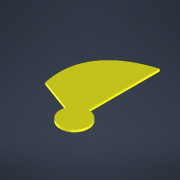
# Autodesk Inventor part: clamshell half
Saved by Autodesk Inventor 2021 (Build 250183000, 183)
## iProperties
Created: 2021-02-13
Part Number: clamshell half
Material: ABS Plastic
Document SubType Name: Modeling
Designer: vikki
Mass: 5.76576 g
Surface Area: 59.2975 cm^2
Volume: 5.43939 cm^3
Density: 1.06 g/cm^3
Appearance: Smooth - Yellow
Author: vikki
Autodesk Inventor part; units mm, degrees
ref_plane "YZ Plane" through (0, 0, 0) normal (1, 0, 0) x (0, 1, 0)
ref_plane "XZ Plane" through (0, 0, 0) normal (0, 1, 0) x (-1, 0, 0)
ref_plane "XY Plane" through (0, 0, 0) normal (0, 0, 1) x (1, 0, 0)
sketch "Sketch1" plane through (0, 0, 0) normal (0, 1, 0) x (-1, 0, 0)
  circle A0 centre (0, 0) radius 12.5
  line L0 (11.7462, -4.2753) -> (40, -14.5588)
  line L1 (0, 0) -> (41.7481, 0) construction
  line L2 (0, 0) -> (11.7462, -4.2753) construction
  line L3 (0, 0) -> (0, -75)
  line L4 (0, -75) -> (27.0598, -66.8927) construction
  line L5 (27.0598, -66.8927) -> (47.507, -49.1207) construction
  line L6 (47.507, -49.1207) -> (40, -14.5588) construction
  spline S0 degree 3 poles (0, -75) (27.0598, -66.8927) (47.507, -49.1207) (40, -14.5588) knots 1 1 1 1 2 2 2 2
  point P0 (0, -12.5)
  dimension "d0" = 25
  dimension "d1" = 40
  dimension "d3" = 20
  dimension "d4" = 75
  constraints: 8 end point, 1 coincident, 1 collinear, 1 horizontal, 1 vertical, 6 other
  measures "d1" horizontal distance of L0.end point (0, 0)
  measures "d3" angle of L1 L0
  measures "d4" distance of L1.start L3.end
extrude "Extrusion1" add sketch "Sketch1" along normal blind 2
sketch "Sketch2" plane through (0, 0, 0) normal (0, -1, 0) x (1, 0, 0)
  circle A0 centre (0, 0) radius 2.5
  dimension "d7" = 5
  constraints: 1 centre point, 1 coincident
  measures "d7" diameter of A0
extrude "Extrusion2" add sketch "Sketch2" along normal blind 4
sketch "Sketch4" plane through (0, 0, 0) normal (0, -1, 0) x (1, 0, 0)
  circle A0 centre (-33.6672, -19.171) radius 1.25 projected
  circle A1 centre (-5, -65) radius 1.25 projected
  point P0 (0, 0)
extrude "Extrusion4" cut sketch "Sketch4" against normal up to surface (2 mm away)
body "Solid1"
